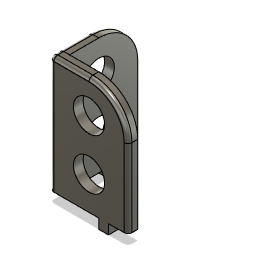
angoli_1.0 (Autodesk Fusion 360 design; units mm, degrees)
Autodesk Fusion 360 part; units mm, degrees
note: some values were not read from the file. Set by a fixed rule: which sketch regions a step uses.
sketch "Sketch5" plane through (0, 0, 0) normal (1, 0, 0) x (0, 0, -1)
  line L0 (25, 0) -> (25, -5)
  line L1 (25, -5) -> (30, -5)
  line L2 (30, -5) -> (30, 0)
  line L3 (30, 0) -> (35, 0)
  line L4 (35, 0) -> (40, 0)
  circle A0 centre (12.5, 2.5) radius 1.5
  circle A1 centre (20, 43) radius 8
  circle A2 centre (20, 17) radius 8
  line L5 (40, 0) -> (40, 40)
  line L6 (20, 60) -> (5, 60)
  arc A3 (40, 40) -> (20, 60) centre (20, 40) ccw
  line L7 (5, 0) -> (5, 60)
  line L8 (25, 0) -> (5, 0)
  dimension "d18" = 3
  dimension "d19" = 20
  constraint perpendicular L0 L1
  constraint perpendicular L1 L2
  constraint perpendicular L0 L3
  constraint perpendicular L0 L4
  constraint perpendicular L4 L5
  constraint tangent L5 A3
  constraint tangent L6 A3
  constraint perpendicular L6 L7
  constraint perpendicular L7 L8
  measures "d18" diameter of A0
  measures "d19" radius of A3
extrude "Extrude6" add sketch "Sketch5" along normal blind 5 makes body 1
sketch "Sketch6" plane through (0, 0, 0) normal (0, 0, 1) x (1, 0, 0)
  line L0 (25, -5) -> (30, -5)
  line L1 (0, 60) -> (0, 0)
  line L2 (30, 0) -> (35, 0)
  arc A0 (40, 40) -> (20, 60) centre (20, 40) ccw
  line L3 (20, 60) -> (0, 60)
  line L4 (35, 0) -> (40, 0)
  circle A1 centre (20, 43) radius 8
  line L5 (0, 0) -> (25, 0)
  line L6 (25, 0) -> (25, -5)
  line L7 (30, -5) -> (30, 0)
  circle A2 centre (20, 17) radius 8
  line L8 (40, 0) -> (40, 40)
  dimension "d21" = 20
  constraint coincident L1.end L5.start
  constraint horizontal L5
  constraint perpendicular L5 L6
  constraint perpendicular L0 L6
  constraint perpendicular L0 L7
  constraint perpendicular L2 L6
  constraint perpendicular L4 L6
  constraint perpendicular L1 L5
  constraint perpendicular L4 L8
  constraint perpendicular L1 L3
  constraint tangent A0 L8
  constraint tangent A0 L3
  measures "d21" radius of A0
extrude "Extrude5" add sketch "Sketch6" against normal blind 5 separate body makes body 2
fillet "Fillet1" radius 2 8 edges at (0, 30, 0) (40, 20, 0) (34.1421, 54.1421, 0) (10, 60, 0) (0, 60, -2.5) (0, 20, -40) (0, 54.1421, -34.1421) (0, 60, -12.5) on bodies 1 2
